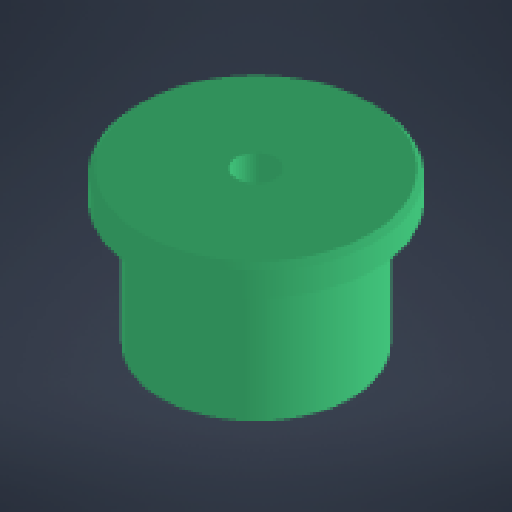
# Autodesk Inventor part: bushing
Saved by Autodesk Inventor 2024 (Build 280153000, 153)
## iProperties
Created: 2023-04-16
Part Number: bushing
Material: Типовые
Document SubType Name: Modeling
Designer: user
Density: 1 g/cm^3
Appearance: По умолчанию
Author: user
Autodesk Inventor part; units mm, degrees
ref_plane "YZ Plane" through (0, 0, 0) normal (1, 0, 0) x (0, 1, 0)
ref_plane "XZ Plane" through (0, 0, 0) normal (0, 1, 0) x (-1, 0, 0)
ref_plane "XY Plane" through (0, 0, 0) normal (0, 0, 1) x (1, 0, 0)
ref_plane "РабПлоскость1" through (19.6828, -0.4261, 0) normal (0, 0, 1) x (0.9982449, -0.0592218, 0)
sketch "Эскиз1" plane through (19.6828, -0.4261, 0) normal (0, 0, 1) x (0.9982449, -0.0592218, 0)
  circle A0 centre (-7.1954, 0) radius 10 projected
  circle A1 centre (-7.1954, 0) radius 12.5 projected
  point P0 (-19.6734, -0.7403)
  point P1 (0.3275, 9.9828)
  point P2 (1.4551, -9.0233)
  point P3 (-15.8459, 9.0233)
  point P4 (-14.7183, -9.9828)
extrude "Выдавливание1" add sketch "Эскиз1" against normal blind 13 contours A0
sketch "Эскиз2" plane through (12.5, 0, 0) normal (0, 0, 1) x (1, 0, 0)
  circle A0 centre (0, 0) radius 12.5 projected
  point P0 (-12.5, 0)
  constraints: 1 horizontal alignment
extrude "Выдавливание2" add sketch "Эскиз2" along normal blind 3
chamfer "Фаска1" distance 0.5 angle 45 1 edges at (0, 0, 3)
sketch "Эскиз3" plane through (12.5, 0, 3) normal (0, 0, 1) x (1, 0, 0)
  circle A0 centre (0, 0) radius 2
  point P0 (-12.5, 0)
  dimension "d7" = 4
  constraints: 1 centre point
  measures "d7" diameter of A0
extrude "Выдавливание3" cut sketch "Эскиз3" against normal through all
sketch "Эскиз4" plane through (12.5, 0, -13) normal (0, 0, -1) x (-1, 0, 0)
  circle A0 centre (0, 0) radius 6
  point P0 (12.5, 0)
  dimension "d10" = 12
  constraints: 1 centre point
  measures "d10" diameter of A0
extrude "Выдавливание4" cut sketch "Эскиз4" against normal blind 13.5
